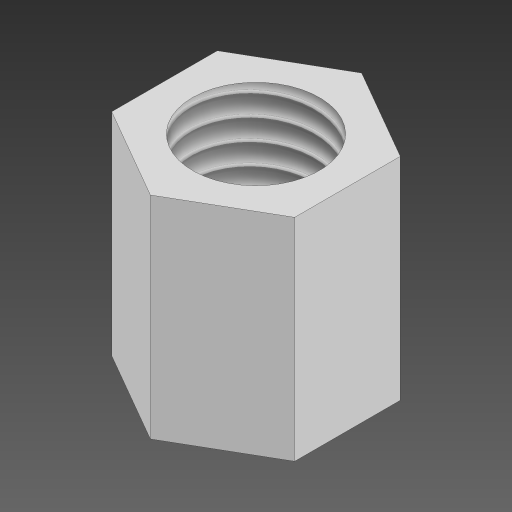
# Autodesk Inventor part: rack_05
Saved by Autodesk Inventor 2023 (Build 270158000, 158)
## iProperties
Created: 2025-07-14
Part Number: rack_05
Material: Типовые
Document SubType Name: Modeling
Designer: daa
Density: 1 g/cm^3
Appearance: По умолчанию
Author: daa
Autodesk Inventor part; units mm, degrees
ref_plane "YZ Plane" through (0, 0, 0) normal (1, 0, 0) x (0, 1, 0)
ref_plane "XZ Plane" through (0, 0, 0) normal (0, 1, 0) x (-1, 0, 0)
ref_plane "XY Plane" through (0, 0, 0) normal (0, 0, 1) x (1, 0, 0)
sketch "Эскиз1" plane through (0, 0, 0) normal (0, 1, 0) x (-1, 0, 0)
  line L0 (0, 3.5153) -> (0, -1.4847)
  line L1 (0, -1.4847) -> (-2.1651, -0.2347)
  line L2 (-2.1651, -0.2347) -> (-2.1651, 2.2653)
  line L3 (-2.1651, 2.2653) -> (0, 3.5153)
  line L4 (0, 3.5153) -> (2.1651, 2.2653)
  line L5 (2.1651, 2.2653) -> (2.1651, -0.2347)
  line L6 (2.1651, -0.2347) -> (0, -1.4847)
  circle A0 centre (0, 1.0153) radius 1.5
  point P0 (0, 0)
  dimension "d0" = 5
  dimension "d1" = 3
  constraints: 14 end point, 1 centre point, 1 coincident, 1 midpoint, 1 vertical, 13 other
  measures "d0" distance of L0.start L0.end
  measures "d1" diameter of A0
extrude "Выдавливание1" add sketch "Эскиз1" along normal blind 5 contours L4 L5 L6 L0 A0 | L0 A0 L1 L2 L3
thread "Резьба1" size "M3x0.5" class "6H" standard "ANSI Metric M Profile" full length
